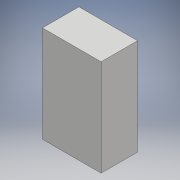
# Autodesk Inventor part: controller_board
Saved by Autodesk Inventor 2018 (Build 220112000, 112)
## iProperties
Created: 2018-02-18
Part Number: controller_board
Material: Generic
Document SubType Name: Modeling
Designer: gaffo
Density: 1 g/cm^3
Appearance: Default
Author: gaffo
Autodesk Inventor part; units mm, degrees
ref_plane "YZ Plane" through (0, 0, 0) normal (1, 0, 0) x (0, 1, 0)
ref_plane "XZ Plane" through (0, 0, 0) normal (0, 1, 0) x (-1, 0, 0)
ref_plane "XY Plane" through (0, 0, 0) normal (0, 0, 1) x (1, 0, 0)
sketch "Sketch1" plane through (0, 0, 0) normal (0, 1, 0) x (-1, 0, 0)
  line L0 (22.5, 37) -> (-22.5, 37)
  line L1 (-22.5, 37) -> (-22.5, -37)
  line L2 (-22.5, -37) -> (22.5, -37)
  line L3 (22.5, -37) -> (22.5, 37)
  point P0 (0, 0)
  point P1 (22.5, 0)
  point P2 (0, -37)
  dimension "d0" = 74
  dimension "d1" = 45
  constraints: 8 end point, 2 midpoint, 2 parallel, 1 horizontal, 1 horizontal alignment, 1 perpendicular, 1 vertical alignment
  measures "d0" distance of L2.end L0.start
  measures "d1" distance of L0.start L0.end
extrude "Extrusion1" add sketch "Sketch1" along normal blind 28
sketch "Sketch2" plane through (-22.5, 0, -37) normal (-1, 0, 0) x (0, 0, 1)
  arc A0 (3, 14) -> (8, 14) centre (5.5, 14) ccw
  arc A1 (8, 21) -> (3, 21) centre (5.5, 21) ccw
  line L0 (8, 14) -> (8, 21)
  line L1 (3, 21) -> (3, 14)
  line L2 (0, 28) -> (74, 28) projected
  line L3 (0, 0) -> (0, 28) projected
  line L4 (37, 0) -> (37, 28) construction
  arc A2 (66, 14) -> (71, 14) centre (68.5, 14) ccw
  arc A3 (71, 21) -> (66, 21) centre (68.5, 21) ccw
  line L5 (66, 14) -> (66, 21)
  line L6 (71, 21) -> (71, 14)
  dimension "d4" = 5
  dimension "d5" = 5
  dimension "d6" = 12
  dimension "d7" = 4.5
  dimension "d8" = 3
  constraints: 10 end point, 8 point on circle, 6 symmetric about line, 4 centre point, 2 tangent, 1 midpoint, 1 parallel, 1 vertical, 2 other
  measures "d4" diameter of A0
  measures "d5" diameter of A1
  measures "d7" distance edge to line of A1 L2
  measures "d8" distance between parallel lines of L3 L1
extrude "Extrusion2" cut sketch "Sketch2" against normal blind 4
equation "\"d5\" = d4"
body "Solid1"
